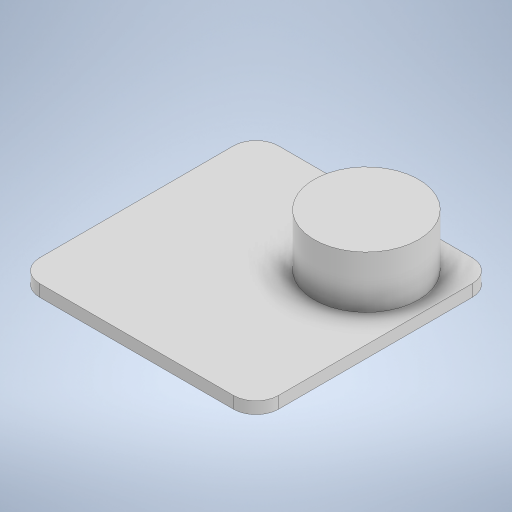
# Autodesk Inventor part: pcb_abs
Saved by Autodesk Inventor 2024 (Build 280153000, 153)
## iProperties
Created: 2023-10-27
Part Number: pcb_abs
Material: 一般
Document SubType Name: Modeling
Designer: Akio
Density: 1 g/cm^3
Appearance: 既定
Author: Akio
Autodesk Inventor part; units mm, degrees
ref_plane "YZ Plane" through (0, 0, 0) normal (1, 0, 0) x (0, 1, 0)
ref_plane "XZ Plane" through (0, 0, 0) normal (0, 1, 0) x (-1, 0, 0)
ref_plane "XY Plane" through (0, 0, 0) normal (0, 0, 1) x (1, 0, 0)
sketch "スケッチ1" plane through (0, 0, 0) normal (0, 1, 0) x (-1, 0, 0)
  line L0 (16, 16) -> (-16, 16)
  line L1 (-16, 16) -> (-16, -16)
  line L2 (-16, -16) -> (16, -16)
  line L3 (16, -16) -> (16, 16)
  line L4 (16, 16) -> (-16, -16) construction
  line L5 (-16, 16) -> (16, -16) construction
  point P0 (0, 0)
  dimension "d0" = 32
  dimension "d1" = 32
  constraints: 12 end point, 2 midpoint, 2 parallel, 1 horizontal, 1 perpendicular
  measures "d0" distance of L2.end L1.end
  measures "d1" distance of L1.end L0.end
extrude "押し出し1" add sketch "スケッチ1" along normal blind 1.6
sketch "スケッチ2" plane through (0, 1.6, 0) normal (0, 1, 0) x (1, 0, 0)
  circle A0 centre (7.3, 7.5) radius 7
  line L0 (16, 16) -> (-16, 16) projected
  line L1 (16, -16) -> (16, 16) projected
  point P0 (0, 0)
  point P1 (13, 16)
  point P2 (-13, 16)
  point P3 (16, -13)
  point P4 (16, 13)
  dimension "d5" = 14
  dimension "d7" = 8.7
  dimension "d8" = 8.5
  constraints: 1 centre point
  measures "d5" diameter of A0
  measures "d7" distance from line of L1 A0.centre
  measures "d8" distance from line of L0 A0.centre
extrude "押し出し2" add sketch "スケッチ2" along normal blind 7
sketch "スケッチ5" plane through (0, 0, 0) normal (0, -1, 0) x (1, 0, 0)
  line L0 (-9, 8) -> (-14, 8)
  line L1 (-14, 8) -> (-14, 1)
  line L2 (-14, 1) -> (-9, 1)
  line L3 (-9, 1) -> (-9, 8)
  line L4 (-9, 8) -> (-14, 1) construction
  line L5 (-14, 8) -> (-9, 1) construction
  line L6 (-16, 16) -> (16, 16) projected
  line L7 (-16, -16) -> (-16, 16) projected
  line L8 (-9, -5) -> (-14, -5)
  line L9 (-14, -5) -> (-14, -12)
  line L10 (-14, -12) -> (-9, -12)
  line L11 (-9, -12) -> (-9, -5)
  line L12 (-9, -5) -> (-14, -12) construction
  line L13 (-14, -5) -> (-9, -12) construction
  point P0 (0, 0)
  point P1 (-11.5, 4.5)
  point P2 (-11.5, -8.5)
  dimension "d19" = 5
  dimension "d20" = 7
  dimension "d21" = 11.5
  dimension "d22" = 4.5
  dimension "d23" = 5
  dimension "d24" = 7
  dimension "d25" = 4.5
  dimension "d26" = 24.5
  constraints: 24 end point, 4 midpoint, 4 parallel, 2 horizontal, 2 perpendicular
  measures "d19" distance of L2.end L1.end
  measures "d20" distance of L1.end L0.end
  measures "d21" distance from line of L6 point (-11.5, 4.5)
  measures "d22" distance from line of L7 point (-11.5, 4.5)
  measures "d23" distance of L10.end L9.end
  measures "d24" distance of L9.end L8.end
  measures "d25" distance from line of L7 point (-11.5, -8.5)
  measures "d26" distance from line of L6 point (-11.5, -8.5)
extrude "押し出し4" add sketch "スケッチ5" along normal blind 2
fillet "フィレット2" radius 3 4 edges at (16, 0.8, -16) (-16, 0.8, -16) (16, 0.8, 16) (-16, 0.8, 16)
